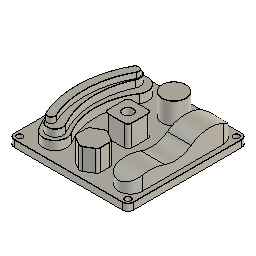
Shapes Target v4 (Autodesk Fusion 360 design; units mm, degrees)
Autodesk Fusion 360 part; units mm, degrees
sketch "Sketch1" plane through (0, 0, 0) normal (0, 0, 1) x (1, 0, 0)
  line L0 (0, 0) -> (150, 0)
  line L1 (150, 0) -> (150, 150)
  line L2 (150, 150) -> (0, 150)
  line L3 (0, 150) -> (0, 0)
  dimension "d1" = 150
  dimension "d2" = 150
  constraint horizontal L0
  constraint vertical L1
  constraint horizontal L2
  constraint vertical L3
  constraint coincident L0.start L3.end
  measures "d1" distance of L0.start L0.end
  measures "d2" distance of L0.start L2.end
extrude "Extrude1" add sketch "Sketch1" along normal blind 9
fillet "Fillet2" radius 7 4 edges at (150, 0, 4.5) (0, 0, 4.5) (0, 150, 4.5) (150, 150, 4.5)
sketch "Sketch4" plane through (0, 0, 0) normal (0, 0, -1) x (1, 0, 0)
  line L0 (0, -7) -> (0, -143)
  line L1 (7, -150) -> (143, -150)
  line L2 (150, -143) -> (150, -7)
  line L3 (143, 0) -> (7, 0)
  line L4 (75, 0) -> (75, -150) construction
  line L5 (0, -75) -> (150, -75) construction
  arc A0 (143, -150) -> (150, -143) centre (143, -143) ccw
  arc A1 (150, -7) -> (143, 0) centre (143, -7) ccw
  arc A2 (7, 0) -> (0, -7) centre (7, -7) ccw
  arc A3 (0, -143) -> (7, -150) centre (7, -143) ccw
  point P0 (24.2, -24.2)
  point P1 (75, -24.2)
  point P2 (125.8, -24.2)
  point P3 (24.2, -75)
  point P4 (75, -75)
  point P5 (125.8, -75)
  point P6 (24.2, -125.8)
  point P7 (75, -125.8)
  point P8 (125.8, -125.8)
  dimension "d7" = 50.8
  dimension "d8" = -50.8
  constraint midpoint L3 L4.start
  constraint midpoint L1 L4.end
  constraint midpoint L0 L5.start
  constraint midpoint L2 L5.end
  constraint symmetric P3 P5 L4
  constraint symmetric P1 P7 L5
sketch "Sketch5" plane through (0, 0, 9) normal (0, 0, 1) x (-1, 0, 0)
  line L0 (0, -143) -> (0, -7)
  line L1 (-7, 0) -> (-143, 0)
  line L2 (-150, -7) -> (-150, -143)
  line L3 (-143, -150) -> (-7, -150)
  line L4 (0, -75) -> (-150, -75)
  line L5 (-75, 0) -> (-75, -150)
  line L6 (-90, -60) -> (-60, -60)
  line L7 (-60, -60) -> (-60, -90)
  line L8 (-60, -90) -> (-90, -90)
  line L9 (-90, -90) -> (-90, -60)
  line L10 (-90, -60) -> (-60, -90) construction
  line L11 (-60, -60) -> (-90, -90) construction
  circle A0 centre (-82, -125.8) radius 15
  line L12 (-97, -32.8603) -> (-82, -41.5205)
  line L13 (-82, -41.5205) -> (-67, -32.8603)
  line L14 (-67, -32.8603) -> (-67, -15.5397)
  line L15 (-67, -15.5397) -> (-82, -6.8795)
  line L16 (-82, -6.8795) -> (-97, -15.5397)
  line L17 (-97, -15.5397) -> (-97, -32.8603)
  arc A1 (-150, -143) -> (-143, -150) centre (-143, -143) ccw
  arc A2 (-7, -150) -> (0, -143) centre (-7, -143) ccw
  arc A3 (0, -7) -> (-7, 0) centre (-7, -7) ccw
  arc A4 (-143, 0) -> (-150, -7) centre (-143, -7) ccw
  line L18 (-24.2, -125.8) -> (-34.2, -125.8)
  line L19 (-24.2, -24.2) -> (-34.2, -24.2)
  line L20 (-24.2, -75) -> (-19.2, -75)
  arc A5 (-21.6059, -133.9479) -> (-21.6059, -16.0521) centre (-112.7213, -75) ccw
  arc A6 (-46.7941, -117.6521) -> (-21.6059, -133.9479) centre (-34.2, -125.8) ccw
  arc A7 (-46.7941, -117.6521) -> (-46.7941, -32.3479) centre (-112.7213, -75) ccw
  arc A8 (-21.6059, -16.0521) -> (-46.7941, -32.3479) centre (-34.2, -24.2) ccw
  arc A9 (-34.2, -125.8) -> (-34.2, -24.2) centre (-112.7213, -75) ccw construction
  line L21 (-125.8, -125.8) -> (-128.8, -125.8)
  line L22 (-125.8, -24.2) -> (-128.8, -24.2)
  line L23 (-113.8, -125.8) -> (-113.8, -24.2)
  arc A10 (-113.8, -24.2) -> (-143.8, -24.2) centre (-128.8, -24.2) ccw
  line L24 (-143.8, -24.2) -> (-143.8, -125.8)
  arc A11 (-143.8, -125.8) -> (-113.8, -125.8) centre (-128.8, -125.8) ccw
  line L25 (-128.8, -125.8) -> (-128.8, -24.2) construction
  line L26 (-75, -125.8) -> (-82, -125.8)
  line L27 (-75, -24.2) -> (-82, -24.2)
  point P0 (-24.2, -125.8)
  point P1 (-75, -125.8)
  point P2 (-125.8, -125.8)
  point P3 (-125.8, -75)
  point P4 (-125.8, -24.2)
  point P5 (-75, -24.2)
  point P6 (-24.2, -24.2)
  point P7 (-24.2, -75)
  point P8 (-75, -75)
  point P9 (-75, -75)
  point P10 (-82, -24.2)
  dimension "d12" = 30
  dimension "d13" = 30
  dimension "d18" = 30
  dimension "d19" = 15
  dimension "d23" = 10
  dimension "d24" = 10
  dimension "d25" = 5
  dimension "d26" = 30
  dimension "d28" = 3
  dimension "d29" = 30
  dimension "d30" = 7
  dimension "d31" = 7
  dimension "d65" = 78.5213
  dimension "d66" = 108.5213
  dimension "d68" = 50.8
  dimension "d69" = 7
  dimension "d70" = 50.8
  dimension "d71" = 136
  dimension "d72" = 150
  dimension "d73" = 50.8
  dimension "d74" = 50.8
  constraint perpendicular L6 L7
  constraint parallel L6 L8
  constraint parallel L7 L9
  constraint horizontal L6
  constraint coincident L10 P9
  constraint coincident L11 P9
  constraint coincident P9 P8
  constraint coincident P0 L18.start
  constraint perpendicular L0 L18
  constraint coincident P6 L19.start
  constraint parallel L4 L19
  constraint coincident P7 L20.start
  constraint parallel L4 L20
  constraint tangent A5 A6
  constraint tangent A6 A7
  constraint tangent A7 A8
  constraint tangent A5 A8
  constraint coincident L18.end A6.centre
  constraint coincident L19.end A8.centre
  constraint parallel L2 L17
  constraint coincident P2 L21.start
  constraint horizontal L21
  constraint coincident P4 L22.start
  constraint horizontal L22
  constraint tangent L23 A10
  constraint tangent A10 L24
  constraint parallel L23 L24
  constraint tangent L24 A11
  constraint tangent L23 A11
  constraint coincident L22.end A10.centre
  constraint perpendicular L22 L25
  constraint coincident L21.end A11.centre
  constraint coincident P1 L26.start
  constraint perpendicular L5 L26
  constraint coincident A0.centre L26.end
  constraint coincident P5 L27.start
  constraint perpendicular L5 L27
  constraint coincident P10 L27.end
  constraint coincident L20.end A9
  measures "d12" distance of L6.start L8.end
  measures "d13" distance of L6.start L6.end
  measures "d18" diameter of A0
  measures "d19" distance of P10 L17
  measures "d23" distance of P0 L18.end
  measures "d24" distance of P6 L19.end
  measures "d25" distance of P7 L20.end
  measures "d26" diameter of A8
  measures "d28" distance of P4 L22.end
  measures "d29" diameter of A10
  measures "d30" distance of P1 A0.centre
  measures "d31" distance of P5 P10
  measures "d65" radius of A7
  measures "d66" radius of A5
  measures "d68" distance of P5 P6
  measures "d69" radius of A1
  measures "d70" distance of P4 P5
  measures "d71" distance of A1.centre A2.centre
  measures "d72" distance of L1 L3
  measures "d73" distance of P9 P1
  measures "d74" distance of P9 P5
extrude "Extrude2" add sketch "Sketch5" along normal blind 27 contours L5 A0 | L5 A0 | L5 L13 L14 L15 | L5 L12 L13 L15 L16 L17 | L4 L5 L8 L9 | L4 L5 L7 L8 | L4 L5 L6 L7 | L4 L5 L6 L9
extrude "Extrude9" add sketch "Sketch5" along normal blind 28 contours L4 L23 A10 L24 | L4 L23 L24 A11
fillet "Fillet1" radius 5 4 edges at (90, 60, 22.5) (60, 60, 22.5) (90, 90, 22.5) (60, 90, 22.5)
fillet "Fillet3" radius 5 6 edges at (67, 15.5397, 22.5) (82, 6.8795, 22.5) (67, 32.8603, 22.5) (82, 41.5205, 22.5) (97, 32.8603, 22.5) (97, 15.5397, 22.5)
hole "Hole2" at (7, 143, 9) at (143, 143, 9) at (143, 7, 9) at (7, 7, 9) direction (0, 0, -1) diameter 7 end up to surface (9 mm away)
sketch "Sketch8" plane through (143.8, 0, 0) normal (1, 0, 0) x (0, 1, 0)
  line L0 (24.2, 8) -> (125.8, 8)
  line L1 (125.8, 8) -> (125.8, 35)
  line L2 (125.8, 35) -> (24.2, 35)
  line L3 (24.2, 35) -> (24.2, 8)
  line L4 (125.8, 21.5) -> (24.2, 21.5) construction
  line L5 (50, 21.5) -> (50, 71.5)
  line L6 (80, 21.5) -> (80, -28.5)
  line L7 (90, 91.5) -> (90, 21.5)
  line L8 (60, 21.5) -> (60, -18.5)
  line L9 (0, 8) -> (50, 71.5)
  line L10 (50, 71.5) -> (60, -18.5)
  line L11 (60, -18.5) -> (80, -28.5)
  line L12 (80, -28.5) -> (90, 91.5)
  line L13 (90, 91.5) -> (150, 8)
  spline S0 degree 5 poles (0, 8) (50, 71.5) (60, -18.5) (80, -28.5) (90, 91.5) (150, 8) knots 0 0 0 0 0 0 1 1 1 1 1 1
  line L14 (0, 8) -> (150, 8)
  line L15 (150, 8) -> (150, 35)
  line L16 (150, 35) -> (0, 35)
  line L17 (0, 35) -> (0, 8)
  point P0 (75, 21.5)
  point P1 (150, 8)
  point P2 (0, 8)
  dimension "d41" = 50
  dimension "d42" = 70
  dimension "d43" = 40
  dimension "d44" = 50
  dimension "d45" = 25
  dimension "d46" = 15
  dimension "d47" = 5
  dimension "d48" = 15
  constraint midpoint L1 L4.start
  constraint midpoint L3 L4.end
  constraint midpoint L4 P0
  constraint coincident L4 L5.start
  constraint perpendicular L4 L5
  constraint perpendicular L4 L6
  constraint coincident L4 L7.end
  constraint perpendicular L4 L7
  constraint coincident L4 L6.start
  constraint coincident L4 L8.start
  constraint perpendicular L4 L8
  constraint coincident P2 L9.start
  constraint coincident L5.end L9.end
  constraint coincident L8.end L10.end
  constraint coincident L6.end L11.end
  constraint coincident L7.start L12.end
  constraint coincident P1 L13.end
  constraint perpendicular L14 L15
  constraint parallel L14 L16
  constraint parallel L15 L17
  constraint collinear L2 L16
  measures "d41" distance of L5.start L5.end
  measures "d42" distance of L7.start L7.end
  measures "d43" distance of L8.start L8.end
  measures "d44" distance of L6.start L6.end
  measures "d45" distance of P0 L5
  measures "d46" distance of P0 L8
  measures "d47" distance of P0 L6
  measures "d48" distance of P0 L7
extrude "Extrude4" [suppressed]
sketch "Side" plane through (143.8, 0, 0) normal (1, 0, 0) x (0, 1, 0)
  line L0 (24.2, 9) -> (125.8, 9)
  line L1 (125.8, 9) -> (125.8, 37)
  line L2 (125.8, 37) -> (24.2, 37)
  line L3 (24.2, 37) -> (24.2, 9)
  line L4 (125.8, 23) -> (24.2, 23) construction
  arc A0 (52.2353, 23.9517) -> (-4.7448, 9) centre (34, -22.6044) ccw
  arc A1 (52.2353, 23.9517) -> (85.5333, 28.197) centre (65, 56.541) ccw
  arc A2 (146.7606, 9) -> (85.5333, 28.197) centre (109, -4.1961) ccw
  line L5 (150, 9) -> (0, 9)
  line L6 (0, 9) -> (0, 37)
  line L7 (0, 37) -> (150, 37)
  line L8 (150, 37) -> (150, 9)
  line L9 (143, 0) -> (143, 9)
  line L10 (143, 9) -> (7, 9)
  line L11 (7, 9) -> (7, 0)
  line L12 (7, 0) -> (143, 0)
  line L13 (143, 9) -> (150, 9)
  line L14 (143, 9) -> (143, 0)
  line L15 (150, 0) -> (143, 0)
  line L16 (150, 0) -> (150, 9)
  line L17 (0, 9) -> (7, 9)
  line L18 (0, 9) -> (0, 0)
  line L19 (7, 0) -> (0, 0)
  line L20 (7, 0) -> (7, 9)
  line L21 (9.2, 9) -> (24.2, 9)
  line L22 (24.2, 9) -> (24.2, 37)
  line L23 (24.2, 37) -> (9.2, 37)
  line L24 (24.2, 37) -> (24.2, 9)
  line L25 (125.8, 9) -> (140.8, 9)
  line L26 (125.8, 9) -> (125.8, 37)
  line L27 (140.8, 37) -> (125.8, 37)
  line L28 (125.8, 37) -> (125.8, 9)
  point P0 (75, 23)
  point P1 (150, 9)
  point P2 (0, 9)
  dimension "d98" = 40
  dimension "d99" = 35
  dimension "d100" = 50
  dimension "d101" = 10
  dimension "d102" = 33.541
  dimension "d103" = 34
  dimension "d104" = 27.1961
  dimension "d105" = 41
  dimension "d106" = 45.6044
  dimension "d109" = 14
  dimension "d110" = 14
  dimension "d111" = 101.6
  dimension "d112" = 50.8
  constraint midpoint L1 L4.start
  constraint midpoint L3 L4.end
  constraint coincident L4 P0
  constraint midpoint L4 P0
  constraint tangent A1 A2
  constraint tangent A0 A1
  constraint coincident L0 A2.start
  constraint coincident L0 A0.end
  constraint coincident P0 A1
  constraint perpendicular L5 L6
  constraint parallel L5 L7
  constraint parallel L6 L8
  constraint coincident P2 L5.end
  constraint parallel L0 L5
  constraint coincident P1 L5.start
  constraint collinear L2 L7
  measures "d98" radius of A2
  measures "d99" radius of A1
  measures "d100" radius of A0
  measures "d101" horizontal distance of P0 A1.centre
  measures "d102" vertical distance of P0 A1.centre
  measures "d103" horizontal distance of P0 A2.centre
  measures "d104" vertical distance of P0 A2.centre
  measures "d105" horizontal distance of P0 A0.centre
  measures "d106" vertical distance of P0 A0.centre
  measures "d109" distance of P0 L5
  measures "d110" distance of L4 L7
  measures "d111" distance of L1 L3
  measures "d112" distance of L4.end P0
extrude "Extrude10" cut sketch "Side" against normal up to surface (30 mm away) contours L3 A0 L6 L7 L22 L23 L24 | L1 L2 L3 A0 A1 A2 L7 L22 L24 L26 L28 | L1 A2 L5 L7 L8 L13 L26 L27 L28
extrude "Extrude5" add sketch "Sketch5" along normal blind 11 contours L4 L20 A5 A6 A7 | L4 L20 A5 A7 A8
sketch "Sketch9" plane through (0, 0, 20) normal (0, 0, 1) x (-1, 0, 0)
  arc A0 (-46.7941, -117.6521) -> (-21.6059, -133.9479) centre (-34.2, -125.8) ccw
  arc A1 (-21.6059, -133.9479) -> (-21.6059, -16.0521) centre (-112.7213, -75) ccw
  arc A2 (-21.6059, -16.0521) -> (-46.7941, -32.3479) centre (-34.2, -24.2) ccw
  arc A3 (-46.7941, -117.6521) -> (-46.7941, -32.3479) centre (-112.7213, -75) ccw
  arc A4 (-34.2, -125.8) -> (-34.2, -24.2) centre (-112.7213, -75) ccw
  line L0 (-34.2, -125.8) -> (-29.2, -125.8)
  arc A5 (-38.28, -121.6103) -> (-42.8248, -29.261) centre (-128.9256, -79.7847) ccw
  arc A6 (-38.28, -121.6103) -> (-20.12, -129.9897) centre (-29.2, -125.8) ccw
  arc A7 (-20.12, -129.9897) -> (-25.5752, -19.139) centre (-128.9256, -79.7847) ccw
  arc A8 (-25.5752, -19.139) -> (-42.8248, -29.261) centre (-34.2, -24.2) ccw
  arc A9 (-29.2, -125.8) -> (-34.2, -24.2) centre (-128.9256, -79.7847) ccw construction
  line L1 (-24.2, -75) -> (-19.2, -75)
  point P0 (-24.2, -125.8)
  point P1 (-24.2, -75)
  point P2 (-24.2, -24.2)
  dimension "d75" = 5
  dimension "d76" = 20
  dimension "d77" = 5
  constraint coincident A0.centre A4.start
  constraint horizontal L0
  constraint tangent A5 A6
  constraint tangent A6 A7
  constraint tangent A7 A8
  constraint tangent A5 A8
  constraint coincident A2.centre A4.end
  constraint coincident L0.end A6.centre
  constraint coincident P1 L1.start
  constraint midpoint A4 L1.end
  constraint coincident A9 L1.end
  measures "d75" distance of A0.centre L0.end
  measures "d76" diameter of A6
  measures "d77" distance of P1 L1.end
extrude "Extrude6" add sketch "Sketch9" along normal blind 9 contours A5 A6 A7 A8
sketch "Sketch11" plane through (0, 0, 29) normal (0, 0, 1) x (-1, 0, 0)
  arc A0 (-38.28, -121.6103) -> (-20.12, -129.9897) centre (-29.2, -125.8) ccw
  arc A1 (-20.12, -129.9897) -> (-25.5752, -19.139) centre (-128.9256, -79.7847) ccw
  arc A2 (-25.5752, -19.139) -> (-42.8248, -29.261) centre (-34.2, -24.2) ccw
  arc A3 (-38.28, -121.6103) -> (-42.8248, -29.261) centre (-128.9256, -79.7847) ccw
  arc A4 (-29.2, -125.8) -> (-34.2, -24.2) centre (-128.9256, -79.7847) ccw
  line L0 (-34.2, -24.2) -> (-29.2, -24.2)
  line L1 (-24.2, -75) -> (-19.2, -75)
  line L2 (-29.2, -125.8) -> (-33.2, -125.8)
  arc A5 (-37.5816, -123.3913) -> (-33.7574, -26.2567) centre (-132.8933, -70.9963) ccw
  arc A6 (-37.5816, -123.3913) -> (-28.8184, -128.2087) centre (-33.2, -125.8) ccw
  arc A7 (-28.8184, -128.2087) -> (-24.6426, -22.1433) centre (-132.8933, -70.9963) ccw
  arc A8 (-24.6426, -22.1433) -> (-33.7574, -26.2567) centre (-29.2, -24.2) ccw
  arc A9 (-33.2, -125.8) -> (-29.2, -24.2) centre (-132.8933, -70.9963) ccw construction
  point P0 (-24.2, -125.8)
  point P1 (-24.2, -24.2)
  point P2 (-24.2, -75)
  dimension "d78" = 5
  dimension "d80" = 5
  dimension "d81" = 5
  dimension "d82" = 5
  dimension "d83" = 4
  dimension "d84" = 10
  constraint coincident A2.centre A4.end
  constraint horizontal L0
  constraint coincident P2 L1.start
  constraint coincident A4 L1.end
  constraint horizontal L1
  constraint coincident A0.centre A4.start
  constraint horizontal L2
  constraint tangent A5 A6
  constraint tangent A6 A7
  constraint tangent A7 A8
  constraint tangent A5 A8
  constraint coincident L0.end A8.centre
  constraint coincident L2.end A6.centre
  measures "d78" distance of A2.centre L0.end
  measures "d80" distance of A0.centre P0
  measures "d81" distance of P1 L0.end
  measures "d82" distance of P2 L1.end
  measures "d83" distance of A0.centre L2.end
  measures "d84" diameter of A6
extrude "Extrude8" add sketch "Sketch11" along normal blind 7 contours A5 A6 A7 A8
sketch "Sketch12" plane through (0, 0, 36) normal (0, 0, 1) x (-1, 0, 0)
  arc A0 (-65, -90) -> (-60, -85) centre (-65, -85) ccw
  line L0 (-60, -85) -> (-60, -65)
  arc A1 (-60, -65) -> (-65, -60) centre (-65, -65) ccw
  line L1 (-65, -60) -> (-85, -60)
  arc A2 (-85, -60) -> (-90, -65) centre (-85, -65) ccw
  line L2 (-90, -65) -> (-90, -85)
  arc A3 (-90, -85) -> (-85, -90) centre (-85, -85) ccw
  line L3 (-85, -90) -> (-65, -90)
  line L4 (-90, -75) -> (-60, -75)
  line L5 (-75, -60) -> (-75, -90)
  point P0 (-75, -75)
  constraint midpoint L2 L4.start
  constraint midpoint L0 L4.end
  constraint midpoint L1 L5.start
  constraint midpoint L3 L5.end
  constraint midpoint L5 P0
hole "Hole3" at (75, 75, 36) direction (0, 0, -1) diameter 12.7 end up to surface (27 mm away)
hole "Hole1" at (24.2, 24.2, 0) at (75, 24.2, 0) at (125.8, 24.2, 0) at (24.2, 75, 0) at (125.8, 75, 0) at (24.2, 125.8, 0) at (75, 125.8, 0) at (125.8, 125.8, 0) direction (0, 0, 1) diameter 5.118 depth 15 tip angle 118
thread "Thread1" "ANSI Unified Screw Threads 0.25 1/4-20 UNC 1B" major diameter 6.35 minor diameter 5.1181 pitch 1.27 angle 60 resizes the face on face at (24.4548, 26.7463, 5) on face at (73.4549, 22.1601, 5) on face at (124.2549, 22.1601, 5) on face at (24.4548, 77.5463, 5) on face at (126.794, 77.3581, 5) on face at (22.0504, 127.1884, 5) on face at (72.8504, 127.1884, 5) on face at (123.6504, 127.1884, 5)
hole "Hole4" at (75, 75, 9) direction (0, 0, -1) diameter 7 end up to surface (9 mm away)
ref_plane "WorkPlane1" through (75, 75, 41) normal (0, 0, 1) x (1, 0, 0)
sketch "Top" plane through (75, 75, 41) normal (0, 0, 1) x (1, 0, 0)
  arc A0 (-28.2059, 42.6521) -> (-28.2059, -42.6521) centre (37.7213, 0) ccw
  arc A1 (-53.3941, -58.9479) -> (-28.2059, -42.6521) centre (-40.8, -50.8) ccw
  arc A2 (-53.3941, 58.9479) -> (-53.3941, -58.9479) centre (37.7213, 0) ccw
  arc A3 (-28.2059, 42.6521) -> (-53.3941, 58.9479) centre (-40.8, 50.8) ccw
  line L0 (68, 75) -> (-68, 75)
  arc A4 (-68, 75) -> (-75, 68) centre (-68, 68) ccw
  line L1 (-75, 68) -> (-75, -68)
  arc A5 (-75, -68) -> (-68, -75) centre (-68, -68) ccw
  line L2 (-68, -75) -> (68, -75)
  arc A6 (68, -75) -> (75, -68) centre (68, -68) ccw
  line L3 (75, -68) -> (75, 68)
  arc A7 (75, 68) -> (68, 75) centre (68, 68) ccw
  circle A8 centre (68, -68) radius 3.5
  circle A9 centre (-68, 68) radius 3.5
  circle A10 centre (68, 68) radius 3.5
  circle A11 centre (-68, -68) radius 3.5
  line L4 (68.8, 50.8) -> (68.8, -50.8)
  arc A12 (38.8, -50.8) -> (68.8, -50.8) centre (53.8, -50.8) ccw
  line L5 (38.8, -50.8) -> (38.8, 50.8)
  arc A13 (68.8, 50.8) -> (38.8, 50.8) centre (53.8, 50.8) ccw
  line L6 (19.5, -60.9036) -> (9.5, -66.6771)
  arc A14 (4.5, -66.6771) -> (9.5, -66.6771) centre (7, -62.347) ccw
  line L7 (4.5, -66.6771) -> (-5.5, -60.9036)
  arc A15 (-8, -56.5735) -> (-5.5, -60.9036) centre (-3, -56.5735) ccw
  line L8 (-8, -56.5735) -> (-8, -45.0265)
  arc A16 (-5.5, -40.6964) -> (-8, -45.0265) centre (-3, -45.0265) ccw
  line L9 (-5.5, -40.6964) -> (4.5, -34.9229)
  arc A17 (9.5, -34.9229) -> (4.5, -34.9229) centre (7, -39.253) ccw
  line L10 (9.5, -34.9229) -> (19.5, -40.6964)
  arc A18 (22, -45.0265) -> (19.5, -40.6964) centre (17, -45.0265) ccw
  line L11 (22, -45.0265) -> (22, -56.5735)
  arc A19 (19.5, -60.9036) -> (22, -56.5735) centre (17, -56.5735) ccw
  circle A20 centre (7, 50.8) radius 15
  line L12 (15, 10) -> (15, -10)
  arc A21 (10, -15) -> (15, -10) centre (10, -10) ccw
  line L13 (10, -15) -> (-10, -15)
  arc A22 (-15, -10) -> (-10, -15) centre (-10, -10) ccw
  line L14 (-15, -10) -> (-15, 10)
  arc A23 (-10, 15) -> (-15, 10) centre (-10, 10) ccw
  line L15 (-10, 15) -> (10, 15)
  arc A24 (15, 10) -> (10, 15) centre (10, 10) ccw
  arc A25 (-37.4184, 48.3913) -> (-41.2426, -48.7433) centre (57.8933, -4.0037) ccw
  arc A26 (-50.3574, -52.8567) -> (-41.2426, -48.7433) centre (-45.8, -50.8) ccw
  arc A27 (-46.1816, 53.2087) -> (-50.3574, -52.8567) centre (57.8933, -4.0037) ccw
  arc A28 (-37.4184, 48.3913) -> (-46.1816, 53.2087) centre (-41.8, 50.8) ccw
  arc A29 (-36.72, 46.6103) -> (-54.88, 54.9897) centre (-45.8, 50.8) ccw
  arc A30 (-54.88, 54.9897) -> (-49.4248, -55.861) centre (53.9256, 4.7847) ccw
  arc A31 (-49.4248, -55.861) -> (-32.1752, -45.739) centre (-40.8, -50.8) ccw
  arc A32 (-36.72, 46.6103) -> (-32.1752, -45.739) centre (53.9256, 4.7847) ccw
  circle A33 centre (0, 0) radius 3.5
  circle A34 centre (0, 0) radius 6.35
chamfer "Chamfer1" distance 0.3 angle 45 60 edges at (95.9849, 131.2242, 36) (88.5355, 61.4645, 36) (90, 75, 36) (88.5355, 88.5355, 36) (75, 90, 36) (61.4645, 88.5355, 36) (60, 75, 36) (61.4645, 61.4645, 36) (75, 60, 36) (69.0797, 77.2963, 36) (82, 40.747, 36) (74.5, 37.1904, 36) (67.6699, 32.4735, 36) (67, 24.2, 36) (67.6699, 15.9265, 36) (74.5, 11.2096, 36) (82, 7.653, 36) (89.5, 11.2096, 36) (96.3301, 15.9265, 36) (97, 24.2, 36) (96.3301, 32.4735, 36) (89.5, 37.1904, 36) (14.2215, 75.6684, 36) (31.2567, 19.6426, 36) (24.2137, 75.2751, 36) (35.6087, 130.1816, 36) (33.3897, 134.88, 29) (9.2406, 73.8947, 29) (39.261, 15.5752, 29) (29.2164, 74.8778, 29) (42.3479, 138.3941, 20) (4.2, 75, 20) (42.3479, 11.6059, 20) (34.2, 75, 20) (147.9497, 2.0503, 9) (150, 75, 9) (147.9497, 147.9497, 9) (75, 150, 9) (2.0503, 147.9497, 9) (0, 75, 9) (2.0503, 2.0503, 9) (75, 0, 9) (150, 75, 0) (147.9497, 147.9497, 0) (75, 150, 0) (2.0503, 147.9497, 0) (0, 75, 0) (2.0503, 2.0503, 0) (75, 0, 0) (147.9497, 2.0503, 0) (139.7369, 8.2657, 9) (3.7369, 8.2657, 9) (3.7369, 144.2657, 9) (139.7369, 144.2657, 9) (71.7369, 73.7343, 0) (139.7369, 141.7343, 0) (3.7369, 141.7343, 0) (3.7369, 5.7343, 0) (139.7369, 5.7343, 0) (71.7369, 76.2657, 9)
fillet "Fillet4" [suppressed]
equation "SmallChamfer = 0.3 mm"
equation "d119 = SmallChamfer"
equation "ToolFillet = 0.2 mm"
equation "d121 = ToolFillet"
